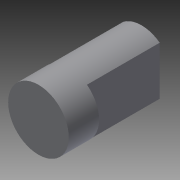
# Autodesk Inventor part: small_stepper_shaft
Saved by Autodesk Inventor 2014 (Build 180170000, 170)
## iProperties
Created: 2015-01-06
Part Number: small_stepper_shaft
Material: Generic
Document SubType Name: Modeling
Designer: cruiser
Density: 1 g/cm^3
Appearance: Default
Author: cruiser
Autodesk Inventor part; units mm, degrees
ref_plane "YZ Plane" through (0, 0, 0) normal (1, 0, 0) x (0, 1, 0)
ref_plane "XZ Plane" through (0, 0, 0) normal (0, 1, 0) x (-1, 0, 0)
ref_plane "XY Plane" through (0, 0, 0) normal (0, 0, 1) x (1, 0, 0)
sketch "Sketch1" plane through (0, 0, 0) normal (0, 1, 0) x (-1, 0, 0)
  circle A0 centre (0, 0) radius 2.5
  dimension "d0" = 5
  constraints: 1 centre point, 1 coincident
  measures "d0" diameter of A0
extrude "Extrusion1" add sketch "Sketch1" along normal blind 2.5
sketch "Sketch2" plane through (0, 2.5, 0) normal (0, 1, 0) x (1, 0, 0)
  circle A0 centre (0, 0) radius 2.5 projected
  line L0 (1.5, -2) -> (-1.5, -2)
  line L1 (-1.5, -2) -> (-1.5, 2)
  line L2 (-1.5, 2) -> (1.5, 2)
  line L3 (1.5, 2) -> (1.5, -2)
  line L4 (1.5, -2) -> (-1.5, 2) construction
  line L5 (-1.5, -2) -> (1.5, 2) construction
  arc A1 (-1.5, -2) -> (1.5, -2) centre (0, 0) ccw
  arc A2 (-1.5, 2) -> (-1.5, -2) centre (0, 0) ccw
  arc A3 (1.5, 2) -> (-1.5, 2) centre (0, 0) ccw
  arc A4 (1.5, -2) -> (1.5, 2) centre (0, 0) ccw
  dimension "d3" = 3
  constraints: 12 end point, 8 point on circle, 4 centre point, 2 midpoint, 2 parallel, 1 coincident, 1 horizontal, 1 perpendicular, 2 other
  measures "d3" distance of L1.end L2.end
extrude "Extrusion2" add sketch "Sketch2" along normal blind 6 contours L2 A0 | L3 L0 L1 L2 | A0 L0
body "Solid1"
